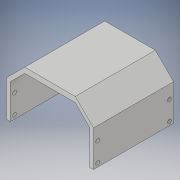
# Autodesk Inventor part: MotorProtector
Saved by Autodesk Inventor 2017 (Build 210142000, 142)
## iProperties
Created: 2017-11-28
Part Number: MotorProtector
Material: Generic
Document SubType Name: Modeling
Designer: User
Density: 1 g/cm^3
Appearance: Default
Author: User
Autodesk Inventor part; units mm, degrees
ref_plane "YZ Plane" through (0, 0, 0) normal (1, 0, 0) x (0, 1, 0)
ref_plane "XZ Plane" through (0, 0, 0) normal (0, 1, 0) x (-1, 0, 0)
ref_plane "XY Plane" through (0, 0, 0) normal (0, 0, 1) x (1, 0, 0)
sketch "Sketch1" plane through (0, 0, 0) normal (1, 0, 0) x (0, 1, 0)
  line L0 (0, 0) -> (45.466, 0)
  line L1 (45.466, 0) -> (45.466, -67.0814)
  line L2 (45.466, -67.0814) -> (0, -67.0814)
  line L3 (0, -67.0814) -> (0, 0)
  dimension "d0" = 45.466
  dimension "d1" = 67.0814
  constraints: 8 end point, 2 parallel, 1 horizontal, 1 perpendicular
  measures "d0" distance of L1.end L2.end
  measures "d1" distance of L0.end L1.end
extrude "Extrusion1" add sketch "Sketch1" along normal blind 72.898
chamfer "Chamfer1" distance 15.24 angle 45 2 edges at (0, 45.466, -33.5407) (72.898, 45.466, -33.5407)
sketch "Sketch2" plane through (0, 0, 0) normal (0, 0, 1) x (1, 0, 0)
  line L0 (57.658, 45.466) -> (72.898, 30.226) projected
  line L1 (15.24, 45.466) -> (57.658, 45.466) projected
  line L2 (0, 30.226) -> (15.24, 45.466) projected
  line L3 (0, 0) -> (0, 30.226) projected
  line L4 (0, 0) -> (72.898, 0) projected
  line L5 (72.898, 30.226) -> (72.898, 0) projected
  line L6 (0, 0) -> (72.898, 0) projected
  line L7 (15.24, 40.9759) -> (57.658, 40.9759)
  line L8 (57.658, 0) -> (15.24, 0)
  line L9 (3.175, 0) -> (69.723, 0)
  line L10 (69.723, 0) -> (69.723, 28.9109)
  line L11 (3.175, 28.9109) -> (3.175, 0)
  line L12 (3.175, 28.9109) -> (15.24, 40.9759)
  line L13 (57.658, 40.9759) -> (69.723, 28.9109)
  dimension "d12" = 3.175
  dimension "d13" = 3.175
  constraints: 14 end point, 2 horizontal, 2 parallel, 2 point on line, 1 perpendicular
  measures "d12" distance between parallel lines of L5 L10
  measures "d13" distance between parallel lines of L3 L11
extrude "Extrusion2" cut sketch "Sketch2" against normal blind 127 contours L4 L11 L12 L7 L13 L10
sketch "Sketch3" plane through (72.898, 0, 0) normal (1, 0, 0) x (0, 0, -1)
  line L0 (0, 30.226) -> (67.0814, 30.226) projected
  line L1 (0, 30.226) -> (0, 0) projected
  line L2 (0, 0) -> (67.0814, 0) projected
  line L3 (67.0814, 0) -> (67.0814, 30.226) projected
  line L4 (3.5179, 3.175) -> (63.5635, 3.175)
  line L5 (63.5635, 3.175) -> (63.5635, 19.177)
  line L6 (63.5635, 19.177) -> (3.5179, 19.177)
  line L7 (3.5179, 19.177) -> (3.5179, 3.175)
  dimension "d16" = 60.0456
  dimension "d17" = 67.0814
  dimension "d18" = 3.5179
  dimension "d19" = 16.002
  dimension "d20" = 30.226
  dimension "d21" = 3.175
  constraints: 8 end point, 2 parallel, 1 horizontal, 1 perpendicular
  measures "d16" distance of L4.start L4.end
  measures "d17" distance of L1.end L2.end
  measures "d18" distance between parallel lines of L1 L7
  measures "d19" distance of L4.end L5.end
  measures "d20" distance of L2.end L0.end
  measures "d21" distance between parallel lines of L2 L4
hole "Hole1" at (72.898, 19.177, -3.5179) at (72.898, 3.175, -3.5179) at (72.898, 19.177, -63.5635) at (72.898, 3.175, -63.5635) direction (-1, 0, 0) diameter 3.175 end through all
equation "\"d18\" = -0.5 * d16 + 0.5 * d17"
body "Solid1"
